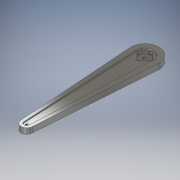
# Autodesk Inventor part: Delta_Arm
Saved by Autodesk Inventor 2019.4 (Build 234330000, 330)
## iProperties
Created: 2019-07-06
Part Number: Delta_Arm
Material: ABS Plastic
Document SubType Name: Modeling
Designer: Jorian Brusind
Density: 1.06 g/cm^3
Appearance: Chrome - Polished
Author: Jorian Brusind
Autodesk Inventor part; units mm, degrees
ref_plane "YZ Plane" through (0, 0, 0) normal (1, 0, 0) x (0, 1, 0)
ref_plane "XZ Plane" through (0, 0, 0) normal (0, 1, 0) x (-1, 0, 0)
ref_plane "Work Plane6" through (0, 10, 0) normal (0, 1, 0) x (1, 0, 0)
sketch "Sketch1" plane through (0, 0, 0) normal (0, 1, 0) x (-1, 0, 0)
  circle A0 centre (0, 0) radius 10
  circle A1 centre (0, -210) radius 25
  line L0 (0, -210) -> (0, 0)
  line L1 (0, 0) -> (10, 0)
  line L2 (0, 0) -> (-10, 0)
  line L3 (0, -210) -> (25, -210)
  line L4 (0, -210) -> (-25, -210)
  line L5 (25, -210) -> (10, 0)
  line L6 (-25, -210) -> (-10, 0)
  point P0 (9.9887, 0.4754)
  dimension "d0" = 20
  dimension "d2" = 50
  dimension "d50" = 210
  dimension "d51" = 210
  constraints: 14 end point, 5 point on circle, 2 centre point, 2 horizontal, 1 coincident, 1 parallel, 1 vertical
  measures "d0" diameter of A0
  measures "d2" diameter of A1
  measures "d50" distance of L0.start point (0, 0)
  measures "d51" vertical distance of L4.end L2.end
ref_plane "Work Plane5" through (0, 10, 0) normal (0, 1, 0) x (1, 0, 0)
ref_plane "Work Plane7" through (0, 10, 0) normal (0, 1, 0) x (1, 0, 0)
ref_plane "Work Plane4" through (0, 0, 0) normal (0, -1, 0) x (1, 0, 0)
ref_plane "Work Plane1" through (0, 5, 0) normal (0, -1, 0) x (1, 0, 0)
ref_plane "Work Plane3" through (0, 10, 0) normal (0, 1, 0) x (1, 0, 0)
ref_plane "Work Plane2" through (0, 0, 5) normal (0, 0, 1) x (1, 0, 0)
extrude "Extrusion8" add sketch "Sketch1" along normal blind 10 contours L1 L2 A0 | L5 A1 L0 A0 | A0 L0 L1 | L2 L0 A0 | A0 L0 A1 L6 | L5 L3 L0 A1 | A1 L0 L4 L6 | A1 L4 L3
sketch "Sketch10" plane through (0, 10, 0) normal (0, 1, 0) x (1, 0, 0)
  circle A0 centre (0, 0) radius 2
  arc A1 (25, 210) -> (-25, 210) centre (0, 210) ccw projected
  circle A2 centre (0, 210) radius 3
  dimension "d54" = 4
  dimension "d55" = 6
  constraints: 2 centre point, 2 coincident
  measures "d54" diameter of A0
  measures "d55" diameter of A2
extrude "Extrusion9" cut sketch "Sketch10" against normal blind 10
sketch "Sketch13" plane through (0, 10, 0) normal (0, 1, 0) x (1, 0, 0)
  arc A0 (-8.9826, 205.2525) -> (-4.6035, 200.9428) centre (0, 210) ccw
  arc A1 (-8.9826, 205.2525) -> (-10.7359, 206.6884) centre (-11.5651, 203.8876) ccw
  arc A2 (-10.7874, 213.1397) -> (-10.7359, 206.6884) centre (-9.7787, 209.9219) ccw
  arc A3 (-3.1397, 199.2126) -> (-4.6035, 200.9428) centre (-5.927, 198.3388) ccw
  arc A4 (-3.1397, 199.2126) -> (3.3116, 199.2641) centre (0.0781, 200.2213) ccw
  arc A5 (4.7475, 201.0174) -> (9.0572, 205.3965) centre (0, 210) ccw
  arc A6 (4.7475, 201.0174) -> (3.3116, 199.2641) centre (6.1124, 198.4349) ccw
  arc A7 (10.7874, 206.8603) -> (10.7359, 213.3116) centre (9.7787, 210.0781) ccw
  arc A8 (8.9826, 214.7475) -> (10.7359, 213.3116) centre (11.5651, 216.1124) ccw
  arc A9 (8.9826, 214.7475) -> (4.6035, 219.0572) centre (0, 210) ccw
  arc A10 (3.1397, 220.7874) -> (4.6035, 219.0572) centre (5.927, 221.6612) ccw
  arc A11 (3.1397, 220.7874) -> (-3.3116, 220.7359) centre (-0.0781, 219.7787) ccw
  arc A12 (-4.7475, 218.9826) -> (-3.3116, 220.7359) centre (-6.1124, 221.5651) ccw
  arc A13 (-4.7475, 218.9826) -> (-9.0572, 214.6035) centre (0, 210) ccw
  arc A14 (-10.7874, 213.1397) -> (-9.0572, 214.6035) centre (-11.6612, 215.927) ccw
  arc A15 (10.7874, 206.8603) -> (9.0572, 205.3965) centre (11.6612, 204.073) ccw
  arc A16 (25, 210) -> (-25, 210) centre (0, 210) ccw projected
  point P0 (0, 0)
  point P1 (-3.2721, -90.998)
  dimension "d63" = 210
  dimension "d64" = 25
  constraints: 32 point on circle, 16 centre point, 4 other
  measures "d63" distance of point (0, 0) A13.centre
  measures "d64" distance of A16.end A16.centre
extrude "Extrusion11" cut sketch "Sketch13" against normal blind 5
ref_plane "Work Plane8" through (0, 5, 0) normal (0, 1, 0) x (1, 0, 0)
sketch "Sketch15" plane through (0, 0, 0) normal (0, -1, 0) x (1, 0, 0)
  circle A0 centre (0, -210) radius 3 projected
  arc A1 (-10.7359, -206.6884) -> (-10.7874, -213.1397) centre (-9.7787, -209.9219) ccw projected
  line L0 (0, -210) -> (-9.7787, -209.9219)
  circle A2 centre (-9.7787, -209.9219) radius 1.5
  point P0 (0, 0)
  dimension "d71" = 3
  constraints: 2 end point, 1 centre point, 1 coincident
  measures "d71" diameter of A2
extrude "Extrusion13" cut sketch "Sketch15" against normal blind 10 contours A2
pattern_circular "Circular Pattern1" count 4 over 360 about axis through (0, 10, -210) along (0, -1, 0) of "Extrusion13"
sketch "Sketch16" plane through (0, 0, 0) normal (0, -1, 0) x (1, 0, 0)
  circle A0 centre (0, -210) radius 3 projected
  circle A1 centre (0, -210) radius 15
  circle A2 centre (0, 0) radius 2 projected
  circle A3 centre (0, 0) radius 5
  line L0 (0, 0) -> (-5, 0)
  line L1 (0, 0) -> (5, 0)
  line L2 (0, -210) -> (-15, -210)
  line L3 (-15, -210) -> (-5, 0)
  line L4 (0, -210) -> (15, -210)
  line L5 (15, -210) -> (5, 0)
  dimension "d77" = 30
  dimension "d78" = 10
  dimension "d79" = 15
  constraints: 12 end point, 3 horizontal, 2 coincident, 2 point on circle, 1 centre point, 1 horizontal alignment, 1 point on line, 2 other
  measures "d78" diameter of A3
  measures "d79" distance of L2.start L2.end
extrude "Extrusion14" cut sketch "Sketch16" against normal blind 2 contours L4 A1 L2 A0 | A0 L2 L3 A1 L5 L4 | L5 A1 | A1 L3 | A1 L3 A3 L5 | L1 A2 L0 A3 | A3 L0 A2 L1 | L1 L0 A2 | A2 L0 L1
mirror "Mirror3" about plane through (0, 5, 0) normal (0, 1, 0) of "Extrusion14"
body "Solid1"
